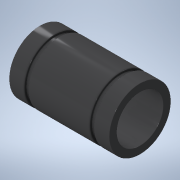
# Autodesk Inventor part: SC8 bearing ext
Saved by Autodesk Inventor 2020.2 (Build 242310000, 310)
## iProperties
Created: 2020-07-09
Part Number: SC8 bearing ext
Material: Ogólny
Document SubType Name: Modeling
Designer: Artur Lenart
Density: 1 g/cm^3
Appearance: PTFE
Author: Artur Lenart
Autodesk Inventor part; units mm, degrees
ref_plane "YZ Plane" through (0, 0, 0) normal (1, 0, 0) x (0, 1, 0)
ref_plane "XZ Plane" through (0, 0, 0) normal (0, 1, 0) x (-1, 0, 0)
ref_plane "XY Plane" through (0, 0, 0) normal (0, 0, 1) x (1, 0, 0)
sketch "Szkic1" plane through (0, 0, 0) normal (1, 0, 0) x (0, 1, 0)
  circle A0 centre (0, 0) radius 8
  circle A1 centre (0, 0) radius 6
  dimension "d0" = 16
  dimension "d1" = 12
  constraints: 2 centre point, 2 coincident
  measures "d0" diameter of A0
  measures "d1" diameter of A1
extrude "Wyciągnięcie proste1" add sketch "Szkic1" along normal blind 26
sketch "Szkic2" plane through (0, 0, 0) normal (0, 0, 1) x (1, 0, 0)
  line L0 (4, 8) -> (5, 8)
  line L1 (5, 8) -> (5, 7.5)
  line L2 (5, 7.5) -> (4, 7.5)
  line L3 (4, 7.5) -> (4, 8)
  line L4 (21, 8) -> (22, 8)
  line L5 (22, 8) -> (22, 7.5)
  line L6 (22, 7.5) -> (21, 7.5)
  line L7 (21, 7.5) -> (21, 8)
  line L8 (26, -8) -> (26, 8) projected
  line L9 (0, -8) -> (0, 8) projected
  line L10 (0, 8) -> (26, 8) projected
  line L11 (-5.2, 0) -> (31.2, 0) projected
  point P0 (0, 0)
  point P1 (4.5, 8)
  point P2 (21.5, 8)
  dimension "d4" = 1
  dimension "d5" = 0.5
  dimension "d6" = 1
  dimension "d7" = 0.5
  dimension "d8" = 4
  dimension "d9" = 4
  constraints: 16 end point, 4 parallel, 2 horizontal, 2 midpoint, 2 perpendicular, 2 point on line
  measures "d4" distance of L1.end L2.end
  measures "d5" distance of L0.end L1.end
  measures "d6" distance of L5.end L6.end
  measures "d7" distance of L4.end L5.end
  measures "d8" distance between parallel lines of L9 L3
  measures "d9" distance between parallel lines of L8 L5
revolve "Obrót1" cut sketch "Szkic2" angle 360 about axis through (-10, 0, 0) along (1, 0, 0) contours L0 L1 L2 L3 | L4 L5 L6 L7
fillet "Zaokrąglenie1" radius 0.1 8 edges at (26, -8, 0) (26, -6, 0) (0, -8, 0) (0, -6, 0) (4, -8, 0) (5, -8, 0) (21, -8, 0) (22, -8, 0)
